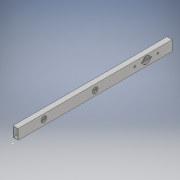
# Autodesk Inventor part: 2x1 20in Alluminum with Cal DropRighttSide.ver1-1111-2019
Saved by Autodesk Inventor 2018 (Build 220112000, 112)
## iProperties
Created: 2019-10-10
Part Number: 2x1 20in Alluminum with Cal DropRighttSide.ver1-1111-2019
Material: Generic
Document SubType Name: Modeling
Designer: JMHal
Density: 1 g/cm^3
Appearance: Default
Author: JMHal
Autodesk Inventor part; units mm, degrees
ref_plane "YZ Plane" through (0, 0, 0) normal (1, 0, 0) x (0, 1, 0)
ref_plane "XZ Plane" through (0, 0, 0) normal (0, 1, 0) x (-1, 0, 0)
ref_plane "XY Plane" through (0, 0, 0) normal (0, 0, 1) x (1, 0, 0)
sketch "Sketch1" plane through (0, 0, 0) normal (0, 1, 0) x (-1, 0, 0)
  point P0 (0, 0)
sketch "Sketch2" plane through (0, 0, 0) normal (0, 1, 0) x (-1, 0, 0)
  line L0 (0, 0) -> (25.4, 0)
  line L1 (25.4, 0) -> (25.4, -812.8)
  line L2 (25.4, -812.8) -> (0, -812.8)
  line L3 (0, -812.8) -> (0, 0)
  dimension "d0" = 812.8
  dimension "d1" = 25.4
  constraints: 8 end point, 2 parallel, 1 horizontal, 1 perpendicular
  measures "d0" distance of L0.end L1.end
  measures "d1" distance of L1.end L2.end
extrude "Extrusion1" add sketch "Sketch2" along normal blind 50.8
sketch "Sketch3" plane through (0, 0, 0) normal (1, 0, 0) x (0, 0, -1)
  circle A0 centre (152.4, 26.9875) radius 14.2875
  line L0 (0, 0) -> (0, 50.8) projected
  line L1 (0, 50.8) -> (812.8, 50.8) projected
  circle A1 centre (660.4, 26.9875) radius 19.05
  line L2 (812.8, 0) -> (812.8, 50.8) projected
  line L3 (812.8, 0) -> (0, 0) projected
  circle A2 centre (406.4, 23.8125) radius 14.2875
  point P0 (406.4, 50.8)
  point P1 (406.4, 0)
  point P2 (406.4, 0)
  dimension "d4" = 28.575
  dimension "d5" = 152.4
  dimension "d6" = 23.8125
  dimension "d7" = 38.1
  dimension "d8" = 152.4
  dimension "d9" = 26.9875
  dimension "d10" = 28.575
  dimension "d11" = 26.9875
  constraints: 3 centre point, 3 midpoint, 3 vertical alignment
  measures "d4" diameter of A0
  measures "d5" distance from line of A0.centre L0
  measures "d6" distance from line of A0.centre L1
  measures "d7" diameter of A1
  measures "d8" distance from line of L2 A1.centre
  measures "d9" distance from line of A1.centre L3
  measures "d10" diameter of A2
  measures "d11" distance from line of A2.centre L1
extrude "Extrusion2" cut sketch "Sketch3" against normal through all contours A0 | A1 | A2
sketch "Sketch4" plane through (-25.4, 0, 0) normal (0, 0, 1) x (1, 0, 0)
  line L0 (0, 50.8) -> (25.4, 50.8) projected
  line L1 (25.4, 0) -> (25.4, 50.8) projected
  line L2 (25.4, 0) -> (0, 0) projected
  line L3 (0, 0) -> (0, 50.8) projected
  line L4 (22.225, 47.625) -> (3.175, 47.625)
  line L5 (3.175, 47.625) -> (3.175, 3.175)
  line L6 (3.175, 3.175) -> (22.225, 3.175)
  line L7 (22.225, 3.175) -> (22.225, 47.625)
  dimension "d15" = 3.175
  constraints: 8 end point, 3 other
  measures "d15" distance between parallel lines of L0 L4
extrude "Extrusion3" cut sketch "Sketch4" against normal up to surface (812.8 mm away) contours L7 L6 L5 L4
sketch "Sketch5" plane through (0, 0, 0) normal (1, 0, 0) x (0, 0, -1)
  circle A0 centre (660.4, 26.9875) radius 19.05 projected
  circle A1 centre (152.4, 26.9875) radius 14.2875 projected
  circle A2 centre (406.4, 23.8125) radius 14.2875 projected
  line L0 (812.8, 0) -> (0, 0) projected
  line L1 (812.8, 0) -> (812.8, 50.8) projected
  line L2 (0, 50.8) -> (812.8, 50.8) projected
  line L3 (0, 0) -> (0, 50.8) projected
  line L4 (0, 50.8) -> (25.4, 50.8)
  line L5 (25.4, 50.8) -> (25.4, 0)
  line L6 (25.4, 0) -> (0, 0)
  line L7 (0, 0) -> (0, 50.8)
  line L8 (812.8, 0) -> (812.8, 50.8) projected
  line L9 (812.8, 0) -> (0, 0) projected
  line L10 (812.8, 50.8) -> (787.4, 50.8)
  line L11 (787.4, 50.8) -> (787.4, 0)
  line L12 (787.4, 0) -> (812.8, 0)
  line L13 (812.8, 0) -> (812.8, 50.8)
  dimension "d18" = 25.4
  dimension "d19" = 25.4
  dimension "d59" = 38.1
  constraints: 16 end point, 4 parallel, 2 horizontal, 2 perpendicular, 2 point on line
  measures "d18" distance between parallel lines of L3 L5
  measures "d19" distance between parallel lines of L1 L11
  measures "d59" diameter of A0
extrude "Extrusion4" cut sketch "Sketch5" against normal blind 25.4 contours L0 L11 L2 L1 | L0 L3 L2 L5
sketch "Sketch6" plane through (0, 0, -25.4) normal (1, 0, 0) x (0, 0, -1)
  line L0 (762, 0) -> (762, 50.8) projected
  circle A0 centre (635, 26.9875) radius 19.05 projected
  line L1 (0, 50.8) -> (762, 50.8) projected
  line L2 (0, 50.8) -> (0, 0) projected
  line L3 (762, 0) -> (0, 0) projected
  line L4 (762, 0) -> (762, 50.8) projected
  line L5 (0, 50.8) -> (762, 50.8) projected
  circle A1 centre (635, 26.9875) radius 19.05 projected
  circle A2 centre (127, 26.9875) radius 14.2875 projected
  circle A3 centre (381, 23.8125) radius 14.2875 projected
  point P0 (-25.4, 0)
  point P1 (658.8125, 26.9875)
  point P2 (611.1875, 26.9875)
  point P3 (692.1754, 26.9875)
  point P4 (577.8246, 26.9875)
  dimension "d37" = 47.625
  dimension "d38" = 23.8125
  dimension "d39" = 57.1754
  dimension "d40" = 57.1754
  dimension "d60" = 38.1
  constraints: 4 horizontal alignment
  measures "d37" distance of point (658.812, 26.988) point (611.187, 26.988)
  measures "d38" distance of A0.centre point (658.812, 26.988)
  measures "d39" distance of point (692.175, 26.988) A0.centre
  measures "d40" distance of point (577.825, 26.988) A0.centre
  measures "d60" diameter of A0
hole "Hole1" at (0, 26.9875, -717.5754) at (0, 26.9875, -603.2246) direction (-1, 0, 0) diameter 4.9784 end through all counterbore diameter 9.525 counterbore depth 6.35
sketch "Sketch7" plane through (0, 0, -25.4) normal (1, 0, 0) x (0, 0, -1)
  circle A0 centre (635, 26.9875) radius 19.05 projected
  point P0 (-25.4, 0)
  point P1 (658.8125, 26.9875)
  point P2 (611.1875, 26.9875)
  dimension "d48" = 47.625
  dimension "d49" = 23.8125
  dimension "d50" = 23.8125
  dimension "d58" = 38.1
  constraints: 1 horizontal alignment
  measures "d48" distance of point (658.812, 26.988) point (611.188, 26.988)
  measures "d49" distance of point (658.812, 26.988) A0.centre
  measures "d50" distance of point (611.188, 26.988) A0.centre
  measures "d58" diameter of A0
hole "Hole2" at (0, 26.9875, -636.5875) at (0, 26.9875, -684.2125) direction (-1, 0, 0) diameter 3.175 end through all counterbore diameter 6.35 counterbore depth 6.35
equation "\"d9\" = d11"
equation "\"d38\" = 0.5 * d37"
equation "\"d40\" = d39"
equation "\"d50\" = d49"
body "Solid1"
